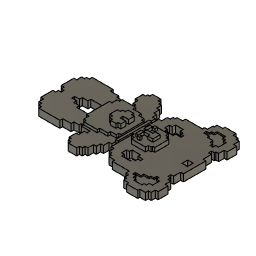
urs breloc varianta cea mai buna v0 (Autodesk Fusion 360 design; units mm, degrees)
Autodesk Fusion 360 part; units mm, degrees
sketch "bear" plane through (0, 0, 0) normal (0, 0, 1) x (1, 0, 0)
  line L0 (55.1506, 25.2183) -> (55.1506, 18.2183)
  line L1 (55.1506, 18.2183) -> (53.1506, 18.2183)
  line L2 (53.1506, 18.2183) -> (53.1506, 14.2183)
  line L3 (53.1506, 14.2183) -> (51.1506, 14.2183)
  line L4 (51.1506, 14.2183) -> (51.1506, 13.2183)
  line L5 (51.1506, 13.2183) -> (49.1506, 13.2183)
  line L6 (49.1506, 13.2183) -> (49.1506, 11.2183)
  line L7 (49.1506, 11.2183) -> (51.1506, 11.2183)
  line L8 (51.1506, 11.2183) -> (51.1506, 5.2183)
  line L9 (51.1506, 5.2183) -> (53.1506, 5.2183)
  line L10 (53.1506, 5.2183) -> (53.1506, -10.7817)
  line L11 (53.1506, -10.7817) -> (51.1506, -10.7817)
  line L12 (51.1506, -10.7817) -> (51.1506, -15.7817)
  line L13 (51.1506, -15.7817) -> (49.1506, -15.7817)
  line L14 (49.1506, -15.7817) -> (49.1506, -17.7817)
  line L15 (49.1506, -17.7817) -> (51.1506, -17.7817)
  line L16 (51.1506, -17.7817) -> (51.1506, -19.7817)
  line L17 (51.1506, -19.7817) -> (53.1506, -19.7817)
  line L18 (53.1506, -23.7817) -> (55.1506, -23.7817)
  line L19 (55.1506, -23.7817) -> (55.1506, -30.7817)
  line L20 (55.1506, -30.7817) -> (53.1506, -30.7817)
  line L21 (53.1506, -19.7817) -> (53.1506, -23.7817)
  line L22 (53.1506, -33.7817) -> (53.1506, -30.7817)
  line L23 (53.1506, -33.7817) -> (51.1506, -33.7817)
  line L24 (51.1506, -33.7817) -> (51.1506, -35.7817)
  line L25 (51.1506, -35.7817) -> (47.1506, -35.7817)
  line L26 (47.1506, -35.7817) -> (47.1506, -37.2608)
  line L27 (47.1506, -37.2608) -> (39.1506, -37.2608)
  line L28 (39.1506, -37.2608) -> (39.1506, -35.7817)
  line L29 (39.1506, -35.7817) -> (35.674, -35.7817)
  line L30 (35.674, -35.7817) -> (35.674, -33.7817)
  line L31 (35.674, -33.7817) -> (34.1506, -33.7817)
  line L32 (34.1506, -33.7817) -> (34.1506, -30.7817)
  line L33 (34.1506, -30.7817) -> (32.1506, -30.7817)
  line L34 (32.1506, -30.7817) -> (32.1506, -28.4279)
  line L35 (32.1506, -28.4279) -> (20.1506, -28.4279)
  line L36 (20.1506, -28.4279) -> (20.1506, -26.7817)
  line L37 (20.1506, -26.7817) -> (16.1506, -26.7817)
  line L38 (16.1506, -26.7817) -> (16.1506, -24.7817)
  line L39 (16.1506, -24.7817) -> (14.5845, -24.7817)
  line L40 (14.5845, -24.7817) -> (14.5845, -23.2754)
  line L41 (14.5845, -23.2754) -> (12.7553, -23.2754)
  line L42 (12.7553, -23.2754) -> (12.7553, -19.8997)
  line L43 (12.7553, -19.8997) -> (10.6351, -19.8997)
  line L44 (10.6351, -19.8997) -> (10.6351, -14.7817)
  line L45 (10.6351, -14.7817) -> (9.1506, -14.7817)
  line L46 (9.1506, -14.7817) -> (9.1506, -17.7817)
  line L47 (9.1506, -17.7817) -> (7.1506, -17.7817)
  line L48 (7.1506, -17.7817) -> (7.1506, -21.7817)
  line L49 (7.1506, -21.7817) -> (5.1506, -21.7817)
  line L50 (5.1506, -21.7817) -> (5.1506, -24.7817)
  line L51 (5.1506, -24.7817) -> (3.1506, -24.7817)
  line L52 (3.1506, -24.7817) -> (3.1506, -28.7817)
  line L53 (3.1506, -28.7817) -> (1.1506, -28.7817)
  line L54 (1.1506, -28.7817) -> (1.1506, -30.7817)
  line L55 (1.1506, -30.7817) -> (-0.8494, -30.7817)
  line L56 (-0.8494, -30.7817) -> (-0.8494, -32.7817)
  line L57 (-0.8494, -32.7817) -> (-6.8494, -32.7817)
  line L58 (-6.8494, -32.7817) -> (-6.8494, -30.7817)
  line L59 (-6.8494, -30.7817) -> (-8.8494, -30.7817)
  line L60 (-8.8494, -30.7817) -> (-8.8494, -28.7817)
  line L61 (-8.8494, -28.7817) -> (-10.2295, -28.7817)
  line L62 (-10.2295, -28.7817) -> (-10.2295, -23.7817)
  line L63 (-10.2295, -23.7817) -> (-8.3918, -23.7817)
  line L64 (-8.3918, -23.7817) -> (-8.3918, -19.7817)
  line L65 (-8.3918, -19.7817) -> (-6.4459, -19.7817)
  line L66 (-6.4459, -19.7817) -> (-6.4459, -17.7817)
  line L67 (-6.4459, -17.7817) -> (-12.4997, -17.7817)
  line L68 (-12.4997, -17.7817) -> (-12.4997, -16.1256)
  line L69 (-12.4997, -16.1256) -> (-14.146, -16.1256)
  line L70 (-14.146, -16.1256) -> (-14.146, -17.7817)
  line L71 (-14.146, -17.7817) -> (-17.8494, -17.7817)
  line L72 (-17.8494, -17.7817) -> (-17.8494, -19.7817)
  line L73 (-17.8494, -19.7817) -> (-23.8494, -19.7817)
  line L74 (-23.8494, -19.7817) -> (-23.8494, -21.7817)
  line L75 (-23.8494, -21.7817) -> (-38.8494, -21.7817)
  line L76 (-38.8494, -21.7817) -> (-38.8494, -19.7817)
  line L77 (-38.8494, -19.7817) -> (-40.8494, -19.7817)
  line L78 (-40.8494, -19.7817) -> (-40.8494, -17.7817)
  line L79 (-40.8494, -17.7817) -> (-42.8494, -17.7817)
  line L80 (-42.8494, -17.7817) -> (-42.8494, -14.3535)
  line L81 (-42.8494, -14.3535) -> (-44.8494, -14.3535)
  line L82 (-44.8494, -14.3535) -> (-44.8494, -5.7817)
  line L83 (-44.8494, -5.7817) -> (-42.8494, -5.7817)
  line L84 (-42.8494, -5.7817) -> (-42.8494, -3.7817)
  line L85 (-42.8494, -3.7817) -> (-40.8494, -3.7817)
  line L86 (-40.8494, -1.7817) -> (-42.8494, -1.7817)
  line L87 (-42.8494, -1.7817) -> (-42.8494, 0.2183)
  line L88 (-42.8494, 0.2183) -> (-44.8494, 0.2183)
  line L89 (-44.8494, 0.2183) -> (-44.8494, 9.2183)
  line L90 (-44.8494, 9.2183) -> (-42.8494, 9.2183)
  line L91 (-42.8494, 9.2183) -> (-42.8494, 12.7535)
  line L92 (-42.8494, 12.7535) -> (-40.8494, 12.7535)
  line L93 (-40.8494, 12.7535) -> (-40.8494, 14.2183)
  line L94 (-40.8494, 14.2183) -> (-38.8494, 14.2183)
  line L95 (-38.8494, 14.2183) -> (-38.8494, 16.2183)
  line L96 (-38.8494, 16.2183) -> (-23.8494, 16.2183)
  line L97 (-23.8494, 16.2183) -> (-23.8494, 14.2183)
  line L98 (-23.8494, 14.2183) -> (-17.8494, 14.2183)
  line L99 (-17.8494, 14.2183) -> (-17.8494, 12.7042)
  line L100 (-17.8494, 12.7042) -> (-14.202, 12.7042)
  line L101 (-14.202, 12.7042) -> (-14.202, 11.2183)
  line L102 (-14.202, 11.2183) -> (-12.5727, 11.2183)
  line L103 (-12.5727, 11.2183) -> (-12.5727, 12.7042)
  line L104 (-12.5727, 12.7042) -> (-6.3757, 12.7042)
  line L105 (-6.3757, 12.7042) -> (-6.3757, 14.6915)
  line L106 (-6.3757, 14.6915) -> (-8.325, 14.6915)
  line L107 (-8.325, 14.6915) -> (-8.325, 18.2183)
  line L108 (-8.325, 18.2183) -> (-10.2743, 18.2183)
  line L109 (-10.2743, 18.2183) -> (-10.2743, 23.7579)
  line L110 (-10.2743, 23.7579) -> (-8.325, 23.7579)
  line L111 (-8.325, 23.7579) -> (-8.325, 25.2183)
  line L112 (-8.325, 25.2183) -> (-6.8494, 25.2183)
  line L113 (-6.8494, 25.2183) -> (-6.8494, 27.2183)
  line L114 (-6.8494, 27.2183) -> (-0.8494, 27.2183)
  line L115 (-0.8494, 27.2183) -> (-0.8494, 25.2183)
  line L116 (-0.8494, 25.2183) -> (1.1506, 25.2183)
  line L117 (1.1506, 25.2183) -> (1.1506, 23.6212)
  line L118 (1.1506, 23.6212) -> (3.1506, 23.6212)
  line L119 (3.1506, 23.6212) -> (3.1506, 20.2183)
  line L120 (3.1506, 20.2183) -> (5.1506, 20.2183)
  line L121 (5.1506, 20.2183) -> (5.1506, 16.2183)
  line L122 (5.1506, 16.2183) -> (7.1506, 16.2183)
  line L123 (7.1506, 16.2183) -> (7.1506, 13.2183)
  line L124 (7.1506, 13.2183) -> (9.1506, 13.2183)
  line L125 (9.1506, 13.2183) -> (9.1506, 9.2183)
  line L126 (9.1506, 9.2183) -> (10.7124, 9.2183)
  line L127 (10.7124, 9.2183) -> (10.7124, 14.2183)
  line L128 (10.7124, 14.2183) -> (12.6538, 14.2183)
  line L129 (12.6538, 14.2183) -> (12.6538, 18.2495)
  line L130 (12.6538, 18.2495) -> (14.616, 18.2495)
  line L131 (14.616, 18.2495) -> (14.616, 20.2183)
  line L132 (14.616, 20.2183) -> (16.1506, 20.2183)
  line L133 (16.1506, 20.2183) -> (16.1506, 21.5941)
  line L134 (16.1506, 21.5941) -> (20.1506, 21.5941)
  line L135 (20.1506, 21.5941) -> (20.1506, 23.69)
  line L136 (20.1506, 23.69) -> (32.1506, 23.69)
  line L137 (32.1506, 23.69) -> (32.1506, 25.2183)
  line L138 (32.1506, 25.2183) -> (34.1506, 25.2183)
  line L139 (34.1506, 25.2183) -> (34.1506, 29.2183)
  line L140 (34.1506, 29.2183) -> (35.1506, 29.2183)
  line L141 (35.1506, 29.2183) -> (35.1506, 31.2183)
  line L142 (35.1506, 31.2183) -> (39.1506, 31.2183)
  line L143 (39.1506, 31.2183) -> (39.1506, 32.7392)
  line L144 (39.1506, 32.7392) -> (47.1506, 32.7392)
  line L145 (47.1506, 32.7392) -> (47.1506, 30.6466)
  line L146 (47.1506, 30.6466) -> (50.6926, 30.6466)
  line L147 (50.6926, 30.6466) -> (50.6926, 29.2183)
  line L148 (50.6926, 29.2183) -> (52.8777, 29.2183)
  line L149 (52.8777, 29.2183) -> (52.8777, 25.2183)
  line L150 (52.8777, 25.2183) -> (55.1506, 25.2183)
  line L151 (-40.8494, -3.7817) -> (-40.8494, -2.7817)
  line L152 (-40.8494, -2.7817) -> (-33.3227, -2.7817)
  line L153 (-33.3227, -3.7817) -> (-29.8494, -3.7817)
  line L154 (-29.8494, -3.7817) -> (-29.8494, -5.7817)
  line L155 (-29.8494, -5.7817) -> (-25.8494, -5.7817)
  line L156 (-25.8494, -5.7817) -> (-25.8494, -7.7817)
  line L157 (-25.8494, -7.7817) -> (-17.8494, -7.7817)
  line L158 (-17.8494, -7.7817) -> (-17.8494, 2.2183)
  line L159 (-17.8494, 2.2183) -> (-25.8494, 2.2183)
  line L160 (-25.8494, 2.2183) -> (-25.8494, 0.2183)
  line L161 (-25.8494, 0.2183) -> (-29.8494, 0.2183)
  line L162 (-29.8494, 0.2183) -> (-29.8494, -1.7817)
  line L163 (-29.8494, -1.7817) -> (-33.3673, -1.7817)
  line L164 (-40.8494, -1.7817) -> (-40.8494, -2.7817)
  line L165 (-33.3673, -1.7817) -> (-33.3227, -2.7817)
  line L166 (-33.3227, -3.7817) -> (-33.3227, -2.7817)
  line L167 (5.1506, 2.2183) -> (3.1506, 2.2183)
  line L168 (3.1506, 2.2183) -> (3.1506, 3.8305)
  line L169 (3.1506, 3.8305) -> (-0.8494, 3.8305)
  line L170 (-0.8494, 3.8305) -> (-0.8494, 1.8833)
  line L171 (-0.8494, 1.8833) -> (-2.8494, 1.8833)
  line L172 (-2.8494, 1.8833) -> (-2.8494, 0.2183)
  line L173 (-2.8494, 0.2183) -> (-4.8494, 0.2183)
  line L174 (-4.8494, 0.2183) -> (-4.8494, -5.2134)
  line L175 (-4.8494, -5.2134) -> (-2.8494, -5.2134)
  line L176 (-2.8494, -5.2134) -> (-2.8494, -7.377)
  line L177 (-2.8494, -7.377) -> (-0.8494, -7.377)
  line L178 (-0.8494, -7.377) -> (-0.8494, -8.7817)
  line L179 (-0.8494, -8.7817) -> (3.1506, -8.7817)
  line L180 (3.1506, -8.7817) -> (3.1506, -7.377)
  line L181 (3.1506, -7.377) -> (5.1506, -7.377)
  line L182 (5.1506, -7.377) -> (5.1506, -3.7817)
  line L183 (5.1506, -3.7817) -> (3.1506, -3.7817)
  line L184 (3.1506, -3.7817) -> (1.1506, -3.7817)
  line L185 (1.1506, -3.7817) -> (1.1506, -1.7817)
  line L186 (1.1506, -1.7817) -> (3.1506, -1.7817)
  line L187 (3.1506, -1.7817) -> (5.1506, -1.7817)
  line L188 (5.1506, -1.7817) -> (5.1506, 2.2183)
  line L189 (29.7264, -17.8185) -> (29.7264, -16.2045)
  line L190 (29.7264, -16.2045) -> (26.1506, -16.2045)
  line L191 (26.1506, -16.2045) -> (26.1506, -14.3953)
  line L192 (26.1506, -14.3953) -> (20.1506, -14.3953)
  line L193 (20.1506, -14.3953) -> (20.1506, -16.2045)
  line L194 (20.1506, -16.2045) -> (18.1506, -16.2045)
  line L195 (18.1506, -16.2045) -> (18.1506, -19.7817)
  line L196 (18.1506, -19.7817) -> (20.1506, -19.7817)
  line L197 (20.1506, -19.7817) -> (20.1506, -21.7817)
  line L198 (20.1506, -21.7817) -> (26.1506, -21.7817)
  line L199 (26.1506, -21.7817) -> (26.1506, -19.7817)
  line L200 (26.1506, -19.7817) -> (27.8497, -19.7817)
  line L201 (27.8497, -19.7817) -> (27.8497, -17.8185)
  line L202 (27.8497, -17.8185) -> (29.7264, -17.8185)
  line L203 (29.7096, 12.8427) -> (27.7275, 12.8427)
  line L204 (27.7275, 12.8427) -> (27.7275, 14.2183)
  line L205 (27.7275, 14.2183) -> (25.7964, 14.2183)
  line L206 (25.7964, 14.2183) -> (25.7964, 16.5209)
  line L207 (25.7964, 16.5209) -> (20.1506, 16.5209)
  line L208 (20.1506, 16.5209) -> (20.1506, 14.2183)
  line L209 (20.1506, 14.2183) -> (18.1506, 14.2183)
  line L210 (18.1506, 14.2183) -> (18.1506, 10.9423)
  line L211 (18.1506, 10.9423) -> (20.1506, 10.9423)
  line L212 (20.1506, 10.9423) -> (20.1506, 9.2183)
  line L213 (20.1506, 9.2183) -> (25.7964, 9.2183)
  line L214 (25.7964, 9.2183) -> (25.7964, 10.9423)
  line L215 (25.7964, 10.9423) -> (29.7096, 10.9423)
  line L216 (29.7096, 10.9423) -> (29.7096, 12.8427)
  line L217 (29.7142, 2.2287) -> (29.7142, -7.7817)
  line L218 (29.7142, -7.7817) -> (28.1506, -7.7817)
  line L219 (28.1506, -7.7817) -> (28.1506, -8.7817)
  line L220 (28.1506, -8.7817) -> (26.1506, -8.7817)
  line L221 (26.1506, -8.7817) -> (26.1506, -10.7817)
  line L222 (26.1506, -10.7817) -> (16.1506, -10.7817)
  line L223 (16.1506, -10.7817) -> (16.1506, -8.7817)
  line L224 (16.1506, -8.7817) -> (14.1506, -8.7817)
  line L225 (14.1506, -8.7817) -> (14.1506, -7.7817)
  line L226 (14.1506, -7.7817) -> (14.1506, -6.7817)
  line L227 (14.1506, -6.7817) -> (12.6148, -6.7817)
  line L228 (12.6148, -6.7817) -> (12.6148, 1.7628)
  line L229 (12.6148, 1.7628) -> (14.1506, 1.7628)
  line L230 (14.1506, 1.7628) -> (14.1506, 3.6195)
  line L231 (14.1506, 3.6195) -> (16.1506, 3.6195)
  line L232 (16.1506, 3.6195) -> (16.1506, 5.5237)
  line L233 (16.1506, 5.5237) -> (26.1506, 5.5237)
  line L234 (26.1506, 5.5237) -> (26.1506, 3.6195)
  line L235 (26.1506, 3.6195) -> (27.8266, 3.6195)
  line L236 (27.8266, 3.6195) -> (27.8266, 2.2183)
  line L237 (27.8266, 2.2183) -> (29.7142, 2.2287)
  line L238 (25.7752, -5.1658) -> (22.1506, -5.1658)
  line L239 (22.1506, -5.1658) -> (22.1506, -3.7817)
  line L240 (22.1506, -3.7817) -> (18.1506, -3.7817)
  line L241 (18.1506, -3.7817) -> (18.1506, -7.2916)
  line L242 (18.1506, -7.2916) -> (20.1506, -7.2916)
  line L243 (20.1506, -7.2916) -> (20.1506, -8.7817)
  line L244 (20.1506, -8.7817) -> (18.1506, -8.7817)
  line L245 (18.1506, -8.7817) -> (18.1506, -7.7817)
  line L246 (18.1506, -7.7817) -> (16.1506, -7.7817)
  line L247 (16.1506, -7.7817) -> (16.1506, -3.7817)
  line L248 (16.1506, -3.7817) -> (17.8728, -3.7817)
  line L249 (17.8728, -3.7817) -> (17.8728, -1.7817)
  line L250 (17.8728, -1.7817) -> (16.1506, -1.7817)
  line L251 (16.1506, -1.7817) -> (16.1506, 2.2183)
  line L252 (16.1506, 2.2183) -> (18.1506, 2.2183)
  line L253 (18.1506, 2.2183) -> (18.1506, 3.7474)
  line L254 (18.1506, 3.7474) -> (20.1506, 3.7474)
  line L255 (20.1506, 3.7474) -> (20.1506, 1.9158)
  line L256 (20.1506, 1.9158) -> (18.1506, 1.9158)
  line L257 (18.1506, 1.9158) -> (18.1506, -1.7817)
  line L258 (18.1506, -1.7817) -> (22.2753, -1.7817)
  line L259 (22.2753, -1.7817) -> (22.2753, 0.067)
  line L260 (22.2753, 0.067) -> (25.7752, 0.067)
  line L261 (25.7752, 0.067) -> (25.7752, -5.1658)
  line L262 (46.8412, -21.8088) -> (46.8412, -23.7817)
  line L263 (46.8412, -23.7817) -> (49.1506, -23.7817)
  line L264 (49.1506, -23.7817) -> (49.1506, -28.7817)
  line L265 (49.1506, -28.7817) -> (46.8412, -28.7817)
  line L266 (46.8412, -28.7817) -> (46.8412, -30.7817)
  line L267 (46.8412, -30.7817) -> (45.1506, -30.7817)
  line L268 (45.1506, -30.7817) -> (45.1506, -32.3666)
  line L269 (45.1506, -32.3666) -> (39.4213, -32.3666)
  line L270 (39.4213, -32.3666) -> (39.4213, -30.7817)
  line L271 (39.4213, -30.7817) -> (37.4298, -30.7817)
  line L272 (37.4298, -30.7817) -> (37.4298, -28.7817)
  line L273 (37.4298, -28.7817) -> (35.1506, -28.7817)
  line L274 (35.1506, -28.7817) -> (35.1506, -27.0988)
  line L275 (35.1506, -27.0988) -> (39.1506, -27.0988)
  line L276 (39.1506, -27.0988) -> (39.1506, -25.0751)
  line L277 (39.1506, -25.0751) -> (42.9546, -25.0751)
  line L278 (42.9546, -25.0751) -> (42.9546, -23.7817)
  line L279 (42.9546, -23.7817) -> (45.1506, -23.7817)
  line L280 (45.1506, -23.7817) -> (45.1506, -21.8088)
  line L281 (45.1506, -21.8088) -> (46.8412, -21.8088)
  line L282 (47.1506, 16.2183) -> (47.1506, 18.2183)
  line L283 (47.1506, 18.2183) -> (49.1506, 18.2183)
  line L284 (49.1506, 18.2183) -> (49.1506, 23.6417)
  line L285 (49.1506, 23.6417) -> (47.1506, 23.6417)
  line L286 (47.1506, 23.6417) -> (47.1506, 25.2183)
  line L287 (47.1506, 25.2183) -> (45.1506, 25.2183)
  line L288 (45.1506, 25.2183) -> (45.1506, 27.2183)
  line L289 (45.1506, 27.2183) -> (39.1506, 27.2183)
  line L290 (39.1506, 27.2183) -> (39.1506, 25.2183)
  line L291 (39.1506, 25.2183) -> (37.1506, 25.2183)
  line L292 (37.1506, 25.2183) -> (37.1506, 23.6417)
  line L293 (37.1506, 23.6417) -> (35.1506, 23.6417)
  line L294 (35.1506, 23.6417) -> (35.1506, 21.5697)
  line L295 (35.1506, 21.5697) -> (39.1506, 21.5697)
  line L296 (39.1506, 21.5697) -> (39.1506, 20.2183)
  line L297 (39.1506, 20.2183) -> (43.1506, 20.2183)
  line L298 (43.1506, 20.2183) -> (43.1506, 18.2183)
  line L299 (43.1506, 18.2183) -> (45.1506, 18.2183)
  line L300 (45.1506, 18.2183) -> (45.1506, 16.2183)
  line L301 (45.1506, 16.2183) -> (47.1506, 16.2183)
  line L302 (9.1506, -14.7817) -> (8.8016, -14.7817)
  line L303 (8.8016, -14.7817) -> (8.8016, 9.2183)
  line L304 (8.8016, 9.2183) -> (9.1506, 9.2183)
  line L305 (10.7124, 9.2183) -> (10.6351, -14.7817)
  line L306 (8.8016, 5.4071) -> (7.1506, 5.4071)
  line L307 (7.1506, 5.4071) -> (7.1506, 7.2183)
  line L308 (7.1506, 7.2183) -> (3.1506, 7.2183)
  line L309 (3.1506, 7.2183) -> (3.1506, 9.2183)
  line L310 (3.1506, 9.2183) -> (-2.8494, 9.2183)
  line L311 (-2.8494, 9.2183) -> (-2.8494, 11.2183)
  line L312 (-2.8494, 11.2183) -> (-12.3933, 11.2183)
  line L313 (-12.3933, 11.2183) -> (-12.3933, 9.2183)
  line L314 (-12.3933, 9.2183) -> (-14.1043, 9.2183)
  line L315 (-14.1043, 9.2183) -> (-14.1043, 5.5563)
  line L316 (-14.1043, 5.5563) -> (-15.8494, 5.5563)
  line L317 (-15.8494, 5.5563) -> (-15.8494, -10.7817)
  line L318 (-15.8494, -10.7817) -> (-14.1043, -10.7817)
  line L319 (-14.1043, -10.7817) -> (-14.1043, -14.4877)
  line L320 (-14.1043, -14.4877) -> (-12.4142, -14.4877)
  line L321 (-12.4142, -14.4877) -> (-12.4142, -16.1337)
  line L322 (-12.4142, -16.1337) -> (-2.8494, -16.1337)
  line L323 (-2.8494, -16.1337) -> (-2.8494, -14.4877)
  line L324 (-2.8494, -14.4877) -> (3.1506, -14.4877)
  line L325 (3.1506, -14.4877) -> (3.1506, -12.6347)
  line L326 (3.1506, -12.6347) -> (7.1506, -12.6347)
  line L327 (7.1506, -12.6347) -> (7.1506, -10.7817)
  line L328 (7.1506, -10.7817) -> (8.8016, -10.7817)
  line L329 (43.1506, 18.2183) -> (43.1506, 20.2183)
  line L330 (50.1506, -0.7817) -> (50.1506, -4.7817)
  line L331 (50.1506, -4.7817) -> (46.1506, -4.7817)
  line L332 (46.1506, -4.7817) -> (46.1506, -0.7817)
  line L333 (46.1506, -0.7817) -> (50.1506, -0.7817)
  dimension "d21" = 16
  dimension "d22" = 70
  constraint perpendicular L0 L1
  constraint perpendicular L1 L2
  constraint perpendicular L2 L3
  constraint perpendicular L3 L4
  constraint perpendicular L4 L5
  constraint perpendicular L5 L6
  constraint perpendicular L4 L7
  constraint perpendicular L7 L8
  constraint perpendicular L8 L9
  constraint perpendicular L9 L10
  constraint perpendicular L10 L11
  constraint perpendicular L9 L12
  constraint perpendicular L12 L13
  constraint perpendicular L9 L14
  constraint perpendicular L12 L15
  constraint perpendicular L15 L16
  constraint perpendicular L16 L17
  constraint perpendicular L16 L18
  constraint perpendicular L18 L19
  constraint perpendicular L19 L20
  constraint perpendicular L18 L21
  constraint perpendicular L20 L22
  constraint perpendicular L22 L23
  constraint perpendicular L20 L24
  constraint perpendicular L24 L25
  constraint perpendicular L23 L26
  constraint perpendicular L26 L27
  constraint perpendicular L27 L28
  constraint perpendicular L28 L29
  constraint perpendicular L29 L30
  constraint perpendicular L30 L31
  constraint perpendicular L31 L32
  constraint perpendicular L32 L33
  constraint perpendicular L33 L34
  constraint perpendicular L32 L35
  constraint perpendicular L33 L36
  constraint perpendicular L36 L37
  constraint perpendicular L37 L38
  constraint perpendicular L38 L39
  constraint perpendicular L39 L40
  constraint perpendicular L40 L41
  constraint perpendicular L41 L42
  constraint perpendicular L42 L43
  constraint perpendicular L43 L44
  constraint perpendicular L44 L45
  constraint perpendicular L45 L46
  constraint perpendicular L46 L47
  constraint perpendicular L45 L48
  constraint perpendicular L48 L49
  constraint perpendicular L49 L50
  constraint perpendicular L50 L51
  constraint perpendicular L49 L52
  constraint perpendicular L52 L53
  constraint perpendicular L49 L54
  constraint perpendicular L52 L55
  constraint perpendicular L55 L56
  constraint perpendicular L56 L57
  constraint perpendicular L57 L58
  constraint perpendicular L58 L59
  constraint perpendicular L59 L60
  constraint perpendicular L60 L61
  constraint perpendicular L59 L62
  constraint perpendicular L62 L63
  constraint perpendicular L59 L64
  constraint perpendicular L64 L65
  constraint perpendicular L65 L66
  constraint perpendicular L66 L67
  constraint perpendicular L67 L68
  constraint perpendicular L68 L69
  constraint perpendicular L69 L70
  constraint perpendicular L70 L71
  constraint perpendicular L71 L72
  constraint perpendicular L70 L73
  constraint perpendicular L71 L74
  constraint perpendicular L74 L75
  constraint perpendicular L75 L76
  constraint perpendicular L76 L77
  constraint perpendicular L77 L78
  constraint perpendicular L78 L79
  constraint perpendicular L79 L80
  constraint perpendicular L80 L81
  constraint perpendicular L81 L82
  constraint perpendicular L80 L83
  constraint perpendicular L81 L84
  constraint perpendicular L84 L85
  constraint perpendicular L86 L87
  constraint perpendicular L87 L88
  constraint perpendicular L86 L89
  constraint perpendicular L87 L90
  constraint perpendicular L90 L91
  constraint perpendicular L87 L92
  constraint perpendicular L92 L93
  constraint perpendicular L87 L94
  constraint perpendicular L92 L95
  constraint perpendicular L95 L96
  constraint perpendicular L92 L97
  constraint perpendicular L97 L98
  constraint perpendicular L98 L99
  constraint perpendicular L97 L100
  constraint perpendicular L100 L101
  constraint perpendicular L97 L102
  constraint perpendicular L100 L103
  constraint perpendicular L97 L104
  constraint perpendicular L104 L105
  constraint perpendicular L105 L106
  constraint perpendicular L106 L107
  constraint perpendicular L105 L108
  constraint perpendicular L108 L109
  constraint perpendicular L109 L110
  constraint perpendicular L110 L111
  constraint perpendicular L111 L112
  constraint perpendicular L110 L113
  constraint perpendicular L111 L114
  constraint perpendicular L114 L115
  constraint perpendicular L115 L116
  constraint perpendicular L116 L117
  constraint perpendicular L117 L118
  constraint perpendicular L118 L119
  constraint perpendicular L119 L120
  constraint perpendicular L120 L121
  constraint perpendicular L119 L122
  constraint perpendicular L122 L123
  constraint perpendicular L119 L124
  constraint perpendicular L122 L125
  constraint perpendicular L119 L126
  constraint perpendicular L126 L127
  constraint perpendicular L127 L128
  constraint perpendicular L126 L129
  constraint perpendicular L129 L130
  constraint perpendicular L130 L131
  constraint perpendicular L129 L132
  constraint perpendicular L132 L133
  constraint perpendicular L129 L134
  constraint perpendicular L134 L135
  constraint perpendicular L135 L136
  constraint perpendicular L136 L137
  constraint perpendicular L135 L138
  constraint perpendicular L138 L139
  constraint perpendicular L139 L140
  constraint perpendicular L138 L141
  constraint perpendicular L139 L142
  constraint perpendicular L142 L143
  constraint perpendicular L143 L144
  constraint perpendicular L144 L145
  constraint perpendicular L145 L146
  constraint perpendicular L146 L147
  constraint perpendicular L145 L148
  constraint perpendicular L146 L149
  constraint perpendicular L0 L150
  constraint perpendicular L85 L151
  constraint perpendicular L151 L152
  constraint perpendicular L152 L154
  constraint perpendicular L154 L155
  constraint perpendicular L155 L156
  constraint perpendicular L154 L157
  constraint perpendicular L155 L158
  constraint perpendicular L158 L159
  constraint perpendicular L155 L160
  constraint perpendicular L160 L161
  constraint perpendicular L161 L162
  constraint perpendicular L162 L163
  constraint perpendicular L152 L164
  constraint perpendicular L152 L166
  constraint perpendicular L167 L168
  constraint perpendicular L168 L169
  constraint perpendicular L169 L170
  constraint perpendicular L170 L171
  constraint perpendicular L169 L172
  constraint perpendicular L172 L173
  constraint perpendicular L169 L174
  constraint perpendicular L174 L175
  constraint perpendicular L175 L176
  constraint perpendicular L174 L177
  constraint perpendicular L177 L178
  constraint perpendicular L178 L179
  constraint perpendicular L177 L180
  constraint perpendicular L180 L181
  constraint perpendicular L177 L182
  constraint perpendicular L180 L183
  constraint perpendicular L180 L184
  constraint perpendicular L184 L185
  constraint perpendicular L185 L186
  constraint perpendicular L185 L187
  constraint perpendicular L167 L188
  constraint perpendicular L189 L190
  constraint perpendicular L190 L191
  constraint perpendicular L189 L192
  constraint perpendicular L190 L193
  constraint perpendicular L193 L194
  constraint perpendicular L194 L195
  constraint perpendicular L193 L196
  constraint perpendicular L196 L197
  constraint perpendicular L197 L198
  constraint perpendicular L196 L199
  constraint perpendicular L199 L200
  constraint perpendicular L196 L201
  constraint perpendicular L201 L202
  constraint perpendicular L203 L204
  constraint perpendicular L204 L205
  constraint perpendicular L205 L206
  constraint perpendicular L206 L207
  constraint perpendicular L205 L208
  constraint perpendicular L206 L209
  constraint perpendicular L205 L210
  constraint perpendicular L206 L211
  constraint perpendicular L211 L212
  constraint perpendicular L206 L213
  constraint perpendicular L211 L214
  constraint perpendicular L206 L215
  constraint perpendicular L203 L216
  constraint perpendicular L217 L218
  constraint perpendicular L218 L219
  constraint perpendicular L219 L220
  constraint perpendicular L220 L221
  constraint perpendicular L219 L222
  constraint perpendicular L222 L223
  constraint perpendicular L223 L224
  constraint perpendicular L224 L225
  constraint perpendicular L224 L226
  constraint perpendicular L226 L227
  constraint perpendicular L227 L228
  constraint perpendicular L228 L229
  constraint perpendicular L229 L230
  constraint perpendicular L228 L231
  constraint perpendicular L229 L232
  constraint perpendicular L232 L233
  constraint perpendicular L233 L234
  constraint perpendicular L234 L235
  constraint perpendicular L235 L236
  constraint perpendicular L217 L238
  constraint perpendicular L238 L239
  constraint perpendicular L239 L240
  constraint perpendicular L238 L241
  constraint perpendicular L241 L242
  constraint perpendicular L242 L243
  constraint perpendicular L243 L244
  constraint perpendicular L242 L245
  constraint perpendicular L245 L246
  constraint perpendicular L246 L247
  constraint perpendicular L247 L248
  constraint perpendicular L246 L249
  constraint perpendicular L249 L250
  constraint perpendicular L250 L251
  constraint perpendicular L251 L252
  constraint perpendicular L252 L253
  constraint perpendicular L253 L254
  constraint perpendicular L254 L255
  constraint perpendicular L255 L256
  constraint perpendicular L254 L257
  constraint perpendicular L255 L258
  constraint perpendicular L254 L259
  constraint perpendicular L259 L260
  constraint perpendicular L260 L261
  constraint perpendicular L262 L263
  constraint perpendicular L263 L264
  constraint perpendicular L264 L265
  constraint perpendicular L263 L266
  constraint perpendicular L266 L267
  constraint perpendicular L267 L268
  constraint perpendicular L268 L269
  constraint perpendicular L269 L270
  constraint perpendicular L270 L271
  constraint perpendicular L271 L272
  constraint perpendicular L272 L273
  constraint perpendicular L273 L274
  constraint perpendicular L274 L275
  constraint perpendicular L273 L276
  constraint perpendicular L274 L277
  constraint perpendicular L273 L278
  constraint perpendicular L274 L279
  constraint perpendicular L273 L280
  constraint perpendicular L280 L281
  constraint perpendicular L144 L282
  constraint perpendicular L282 L283
  constraint perpendicular L144 L284
  constraint perpendicular L284 L285
  constraint perpendicular L285 L286
  constraint perpendicular L284 L287
  constraint perpendicular L287 L288
  constraint perpendicular L284 L289
  constraint perpendicular L287 L290
  constraint perpendicular L290 L291
  constraint perpendicular L287 L292
  constraint perpendicular L292 L293
  constraint perpendicular L287 L294
  constraint perpendicular L292 L295
  constraint perpendicular L295 L296
  constraint perpendicular L292 L297
  constraint perpendicular L297 L298
  constraint perpendicular L292 L299
  constraint perpendicular L299 L300
  constraint perpendicular L282 L301
  constraint perpendicular L46 L302
  constraint perpendicular L126 L303
  constraint perpendicular L125 L304
  constraint coincident L303 L306.start
  constraint perpendicular L303 L306
  constraint perpendicular L306 L307
  constraint perpendicular L303 L308
  constraint perpendicular L308 L309
  constraint perpendicular L303 L310
  constraint perpendicular L310 L311
  constraint perpendicular L311 L312
  constraint perpendicular L312 L313
  constraint perpendicular L311 L314
  constraint perpendicular L314 L315
  constraint perpendicular L315 L316
  constraint perpendicular L314 L317
  constraint perpendicular L317 L318
  constraint perpendicular L318 L319
  constraint perpendicular L319 L320
  constraint perpendicular L320 L321
  constraint perpendicular L319 L322
  constraint perpendicular L320 L323
  constraint perpendicular L323 L324
  constraint perpendicular L320 L325
  constraint perpendicular L323 L326
  constraint perpendicular L320 L327
  constraint coincident L303 L328.end
  constraint perpendicular L303 L328
  constraint perpendicular L9 L330
  constraint perpendicular L330 L331
  constraint perpendicular L331 L332
  constraint perpendicular L330 L333
  measures "d21" distance of L9.end L10.end
  measures "d22" distance of L26.end L144.end
extrude "Extrude1" add sketch "bear" along normal blind 5 contours L0 L1 L2 L3 L4 L5 L6 L7 L8 L9 L10 L11 L12 L13 L14 L15 L16 L17 L18 L19 L20 L21 L22 L23 L24 L25 L26 L27 L28 L29 L30 L31 L32 L33 L34 L35 L36 L37 L38 L39 L40 L41 L42 L43 L44 L127 L128 L129 L130 L131 L132 L133 L134 L135 L136 L137 L138 L139 L140 L141 L142 L143 L144 L145 L146 L147 L148 L149 L150 L305 | L46 L47 L48 L49 L50 L51 L52 L53 L54 L55 L56 L57 L58 L59 L60 L61 L62 L63 L64 L65 L66 L67 L68 L69 L70 L71 L72 L73 L74 L75 L76 L77 L78 L79 L80 L81 L82 L83 L84 L85 L86 L87 L88 L89 L90 L91 L92 L93 L94 L95 L96 L97 L98 L99 L100 L101 L102 L103 L104 L105 L106 L107 L108 L109 L110 L111 L112 L113 L114 L115 L116 L117 L118 L119 L120 L121 L122 L123 L124 L125 L151 L164 L302 L303 L304 L306 L307 L308 L309 L310 L311 L312 L313 L314 L315 L316 L317 L318 L319 L320 L321 L322 L323 L324 L325 L326 L327 L328 makes body 1 at (41.6703, 7.1263, 0) makes body 2 at (-29.5161, 10.2183, 0)
extrude "Extrude2" add sketch "bear" along normal blind 8 separate body contours L217 L218 L219 L220 L221 L222 L223 L224 L225 L226 L227 L228 L229 L230 L231 L232 L233 L234 L235 L236 L237 makes body 3
extrude "Extrude3" add sketch "bear" along normal blind 10 separate body contours L238 L239 L240 L241 L242 L243 L244 L245 L246 L247 L248 L249 L250 L251 L252 L253 L254 L255 L256 L257 L258 L259 L260 L261 makes body 4
extrude "Extrude4" add sketch "bear" along normal blind 7 separate body contours L303 L306 L307 L308 L309 L310 L311 L312 L313 L314 L315 L316 L317 L318 L319 L320 L321 L322 L323 L324 L325 L326 L327 L328 makes body 5
extrude "Extrude5" add sketch "bear" along normal blind 10 separate body contours L167 L168 L169 L170 L171 L172 L173 L174 L175 L176 L177 L178 L179 L180 L181 L182 L183 L184 L185 L186 L187 L188 makes body 6
extrude "Extrude6" add sketch "bear" along normal blind 4 separate body contours L262 L263 L264 L265 L266 L267 L268 L269 L270 L271 L272 L273 L274 L275 L276 L277 L278 L279 L280 L281 | L282 L283 L284 L285 L286 L287 L288 L289 L290 L291 L292 L293 L294 L295 L296 L297 L298 L299 L300 L301 L329 makes body 7 at (42.4186, -27.6519, 0) makes body 8 at (42.4839, 23.5516, 0)
extrude "Extrude7" add sketch "bear" along normal blind 6 contours L45 L126 L302 L303 L304 L305 bodies 2 3 4 6 7 8 1 5
combine "Combine1" operation add target body 2 tool bodies 3 4 6 7 8
named bodies: "bear breloc bun"
